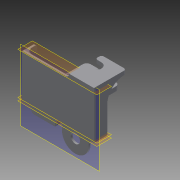
# Autodesk Inventor part: servo-holder
Saved by Autodesk Inventor 2014 (Build 180170000, 170)
## iProperties
Created: 2015-03-09
Part Number: servo-holder
Material: 一般
Document SubType Name: Modeling
Designer: Hideyuki Takei
Density: 1 g/cm^3
Appearance: 既定
Author: Hideyuki Takei
Autodesk Inventor part; units mm, degrees
ref_plane "YZ Plane" through (0, 0, 0) normal (1, 0, 0) x (0, 1, 0)
sketch "スケッチ2" plane through (0, 0, 0) normal (0, 1, 0) x (-1, 0, 0)
  line L0 (-8.8, 25.8) -> (27, 25.8)
  line L1 (27, 25.8) -> (27, 3.8)
  line L2 (27, 3.8) -> (-8.8, 3.8)
  line L3 (-8.8, 3.8) -> (-8.8, 25.8)
  line L4 (-8.8, 25.8) -> (-9.8, 25.8)
  line L5 (-9.8, 25.8) -> (-9.8, 3.8)
  line L6 (-9.8, 3.8) -> (-8.8, 3.8)
  line L7 (-8.8, 3.8) -> (-8.8, 25.8)
  line L8 (27, 25.8) -> (28, 25.8)
  line L9 (28, 25.8) -> (28, 3.8)
  line L10 (28, 3.8) -> (27, 3.8)
  line L11 (27, 3.8) -> (27, 25.8)
  point P0 (0, 0)
  dimension "d3" = 3.8
  dimension "d4" = 8.8
  dimension "d5" = 35.8
  dimension "d6" = 22
  dimension "d7" = 1
  dimension "d8" = 1
  dimension "d9" = 22
  dimension "d10" = 22
  constraints: 24 end point, 6 parallel, 3 horizontal, 3 perpendicular
  measures "d3" distance from line of point (0, 0) L2
  measures "d4" distance from line of point (0, 0) L3
  measures "d5" distance of L0.start L0.end
  measures "d6" distance of L2.end L0.start
  measures "d7" distance of L0.start L4.end
  measures "d8" distance of L0.end L8.end
  measures "d9" distance of L8.end L9.end
  measures "d10" distance of L4.end L5.end
extrude "押し出し2" add sketch "スケッチ2" along normal blind 7
ref_plane "作業平面4" through (0, 1, 0) normal (0, 1, 0) x (-1, 0, 0)
sketch "スケッチ3" plane through (0, 1, 0) normal (0, 1, 0) x (-1, 0, 0)
  line L0 (-8.8, 3.8) -> (27, 3.8)
  line L1 (27, 3.8) -> (27, 25.8)
  line L2 (27, 25.8) -> (-8.8, 25.8)
  line L3 (-8.8, 25.8) -> (-8.8, 3.8)
  point P0 (0, 0)
  dimension "d15" = 22
  dimension "d16" = 35.8
  dimension "d17" = 8.8
  dimension "d18" = 3.8
  constraints: 8 end point, 2 parallel, 1 horizontal, 1 perpendicular
  measures "d15" distance of L2.end L0.start
  measures "d16" distance of L1.end L2.end
  measures "d17" distance from line of point (0, 0) L3
  measures "d18" distance from line of point (0, 0) L0
extrude "押し出し3" cut sketch "スケッチ3" along normal up to next
fillet "フィレット3" radius 5 1 edges at (8.8, 1, 14.8)
sketch "スケッチ1" plane through (0, 0, 0) normal (0, 1, 0) x (-1, 0, 0)
  circle A0 centre (0, 0) radius 7
  dimension "d0" = 14
  constraints: 1 centre point, 1 coincident
  measures "d0" diameter of A0
extrude "押し出し1" add sketch "スケッチ1" along normal blind 1
fillet "フィレット4" radius 3 1 edges at (-27, 1, 14.8)
ref_plane "作業平面5" through (0, 0, 3.8) normal (0, 0, 1) x (1, 0, 0)
sketch "スケッチ4" plane through (0, 0, 3.8) normal (0, 0, 1) x (1, 0, 0)
  circle A0 centre (6.2, 3.6) radius 0.9
  line L0 (-7, 0) -> (7, 0) projected
  circle A1 centre (-24.9, 3.6) radius 0.9
  line L1 (9.8, 7) -> (4.3, 7)
  line L2 (4.3, 7) -> (4.3, 0)
  line L3 (4.3, 0) -> (9.8, 0)
  line L4 (9.8, 0) -> (9.8, 7)
  line L5 (9.8, 0) -> (9.8, 7) projected
  line L6 (-28, 7) -> (-22.7, 7)
  line L7 (-22.7, 7) -> (-22.7, 0)
  line L8 (-22.7, 0) -> (-28, 0)
  line L9 (-28, 0) -> (-28, 7)
  line L10 (-28, 0) -> (-28, 7) projected
  line L11 (-5.8788, 0) -> (-28, 0) projected
  point P0 (0, 0)
  point P1 (5.8788, 0)
  dimension "d27" = 3.6
  dimension "d28" = 6.2
  dimension "d29" = 1.8
  dimension "d30" = 1.8
  dimension "d31" = 3.6
  dimension "d32" = 24.9
  dimension "d33" = 5.5
  dimension "d34" = 7
  dimension "d35" = 0
  dimension "d36" = 0
  dimension "d37" = 5.3
  dimension "d38" = 0
  dimension "d39" = 0
  dimension "d40" = 7
  constraints: 16 end point, 4 parallel, 2 centre point, 2 horizontal, 2 perpendicular
  measures "d27" distance from line of L0 A0.centre
  measures "d28" horizontal distance of point (0, 0) A0.centre
  measures "d29" diameter of A0
  measures "d30" diameter of A1
  measures "d31" vertical distance of point (0, 0) A1.centre
  measures "d32" horizontal distance of A1.centre point (0, 0)
  measures "d33" distance of L1.start L1.end
  measures "d34" distance of L1.end L2.end
  measures "d35" distance between parallel lines of L0 L3
  measures "d36" distance between parallel lines of L5 L4
  measures "d37" distance of L6.start L6.end
  measures "d38" distance between parallel lines of L10 L9
  measures "d39" distance between parallel lines of L11 L8
  measures "d40" distance of L6.end L7.end
extrude "押し出し4" add sketch "スケッチ4" against normal blind 1
ref_plane "作業平面7" through (0, 0, 25.8) normal (0, 0, 1) x (1, 0, 0)
sketch "スケッチ6" plane through (0, 0, 25.8) normal (0, 0, 1) x (1, 0, 0)
  line L0 (9.8, 0) -> (-3.2, 0)
  line L1 (-3.2, 0) -> (-3.2, 17)
  line L2 (-3.2, 17) -> (9.8, 17)
  line L3 (9.8, 17) -> (9.8, 0)
  line L4 (9.8, 0) -> (9.8, 7) projected
  line L5 (-28, 0) -> (9.8, 0) projected
  circle A0 centre (0, 10.8) radius 2.9
  line L6 (0, 13.7) -> (-5.7401, 13.7)
  line L7 (-5.7401, 13.7) -> (-5.7401, 7.9)
  line L8 (-5.7401, 7.9) -> (0, 7.9)
  line L9 (0, 7.9) -> (0, 13.7)
  point P0 (0, 0)
  dimension "d58" = 5.8
  dimension "d54" = 0
  dimension "d55" = 0
  dimension "d56" = 13
  dimension "d57" = 17
  dimension "d59" = 9.8
  dimension "d60" = 10.8
  dimension "d61" = 5.8
  dimension "d62" = 2.9
  dimension "d63" = 5.7401
  constraints: 16 end point, 4 parallel, 2 horizontal, 2 perpendicular, 1 vertical alignment, 2 other
  measures "d54" distance between parallel lines of L4 L3
  measures "d55" distance between parallel lines of L5 L0
  measures "d56" distance of L1.end L2.end
  measures "d57" distance of L2.end L0.start
  measures "d59" distance from line of L3 point (0, 10.8)
  measures "d60" distance from line of L0 point (0, 10.8)
  measures "d61" distance of L6.end L7.end
  measures "d62" distance from line of L8 point (0, 10.8)
  measures "d63" distance of L6.start L6.end
extrude "押し出し5" add sketch "スケッチ6" along normal blind 2 contours L0 L1 L8 A0 L6 L2 L3 | L1 L6 A0 L8
sketch "スケッチ7" plane through (0, 0, 25.8) normal (0, 0, 1) x (1, 0, 0)
  line L0 (0, 13.7) -> (-9.1376, 13.7)
  line L1 (-9.1376, 13.7) -> (-9.1376, 7.9)
  line L2 (-9.1376, 7.9) -> (0, 7.9)
  line L3 (0, 7.9) -> (0, 13.7)
  line L4 (-3.2, 0) -> (9.8, 0) projected
  point P0 (0, 0)
  dimension "d66" = 5.8
  dimension "d67" = 7.9
  dimension "d68" = 0
  dimension "d69" = 9.1376
  constraints: 8 end point, 2 parallel, 1 horizontal, 1 perpendicular
  measures "d66" distance of L0.end L1.end
  measures "d67" distance between parallel lines of L4 L2
  measures "d68" distance from line of point (0, 0) L3
  measures "d69" distance of L0.start L0.end
extrude "押し出し6" cut sketch "スケッチ7" along normal blind 2
fillet "フィレット5" radius 3 1 edges at (4.3, 7, 3.3)
fillet "フィレット6" radius 1.2 5 edges at (-3.2, 17, 26.8) (-3.2, 13.7, 26.8) (9.8, 17, 26.8) (-3.2, 7.9, 26.8) (-27.5, 7, 25.8)
fillet "フィレット7" radius 2 1 edges at (-3.2, 0.5, 25.8)
fillet "フィレット8" radius 2 3 edges at (4.3, 1, 3.3) (-5.8788, 0.5, 3.8) (6.4156, 0.5, 2.8)
sketch "スケッチ8" plane through (0, 1, 0) normal (0, 1, 0) x (-1, 0, 0)
  circle A0 centre (0, 0) radius 2.5
  dimension "d76" = 5
  constraints: 1 centre point, 1 coincident
  measures "d76" diameter of A0
extrude "押し出し7" cut sketch "スケッチ8" against normal up to next
ref_plane "作業平面8" through (0, 0, 2.3) normal (0, 0, 1) x (1, 0, 0)
sketch "スケッチ9" plane through (0, 0, 2.3) normal (0, 0, 1) x (1, 0, 0)
  line L0 (-10.7, 34) -> (-22.7, 34)
  line L1 (-22.7, 34) -> (-22.7, 0)
  line L2 (-22.7, 0) -> (-10.7, 0)
  line L3 (-10.7, 0) -> (-10.7, 34)
  line L4 (-8.8182, 0) -> (-22.7, 0) projected
  line L5 (-22.7, 7) -> (-22.7, 0) projected
  point P0 (0, 0)
  dimension "d80" = 0
  dimension "d81" = 0
  dimension "d82" = 34
  dimension "d83" = 12
  constraints: 8 end point, 2 parallel, 1 horizontal, 1 perpendicular
  measures "d80" distance between parallel lines of L4 L2
  measures "d81" distance between parallel lines of L5 L1
  measures "d82" distance of L2.end L0.start
  measures "d83" distance of L0.start L0.end
extrude "押し出し8" add sketch "スケッチ9" against normal blind 2.3
sketch "スケッチ10" plane through (0, 0, 2.3) normal (0, 0, 1) x (1, 0, 0)
  line L0 (-10.7, 1) -> (-22.7, 1)
  line L1 (-22.7, 1) -> (-22.7, 0)
  line L2 (-22.7, 0) -> (-10.7, 0)
  line L3 (-10.7, 0) -> (-10.7, 1)
  line L4 (-10.7, 34) -> (-10.7, 0) projected
  line L5 (-10.7, 0) -> (-22.7, 0) projected
  point P0 (0, 0)
  dimension "d86" = 1
  dimension "d87" = 12
  dimension "d88" = 0
  dimension "d89" = 0
  constraints: 8 end point, 2 parallel, 1 horizontal, 1 perpendicular
  measures "d86" distance of L2.end L0.start
  measures "d87" distance of L1.end L2.end
  measures "d88" distance between parallel lines of L4 L3
  measures "d89" distance between parallel lines of L5 L2
extrude "押し出し9" add sketch "スケッチ10" along normal up to next
sketch "スケッチ11" plane through (0, 0, 3.8) normal (0, 0, 1) x (1, 0, 0)
  line L0 (-22.7, 34) -> (-28, 34)
  line L1 (-28, 34) -> (-28, 7)
  line L2 (-28, 7) -> (-22.7, 7)
  line L3 (-22.7, 7) -> (-22.7, 34)
  line L4 (-22.7, 1) -> (-22.7, 0) projected
  line L5 (-28, 0) -> (-28, 7) projected
  line L6 (-28, 7) -> (-22.7, 7) projected
  line L7 (-22.7, 34) -> (-10.7, 34) projected
  point P0 (0, 0)
  dimension "d93" = 0
  dimension "d94" = 0
  dimension "d95" = 0
  dimension "d108" = 5.3
  constraints: 8 end point, 2 parallel, 1 horizontal, 1 perpendicular
  measures "d93" distance between parallel lines of L5 L1
  measures "d94" distance between parallel lines of L6 L2
  measures "d95" distance between parallel lines of L7 L0
  measures "d108" distance between parallel lines of L1 L3
extrude "押し出し10" add sketch "スケッチ11" against normal blind 1
sketch "スケッチ12" plane through (0, 0, 2.8) normal (0, 0, -1) x (-1, 0, 0)
  line L0 (22.7, 34) -> (22.7, 0) projected
  line L1 (22.7, 1) -> (22.7, 0) projected
  line L2 (22.7, 0) -> (28, 0) projected
  line L3 (22.7, 34) -> (23.2, 34)
  line L4 (23.2, 34) -> (23.2, 0)
  line L5 (23.2, 0) -> (22.7, 0)
  line L6 (22.7, 0) -> (22.7, 34)
  point P0 (0, 0)
  dimension "d98" = 0.5
  constraints: 8 end point, 2 parallel, 1 horizontal, 1 perpendicular, 1 point on line
  measures "d98" distance of L0.start L3.end
extrude "押し出し11" add sketch "スケッチ12" along normal blind 2.8
fillet "フィレット13" radius 1.5 2 edges at (-23.2, 17, 0) (-23.2, 17, 2.8)
fillet "フィレット9" radius 19 1 edges at (-27.5, 7, 3.8)
sketch "スケッチ13" plane through (0, 0, 2.8) normal (0, 0, -1) x (-1, 0, 0)
  arc A0 (24, 3.6) -> (24, 3.6) centre (24.9, 3.6) ccw projected
  circle A1 centre (24.9, 3.6) radius 1.6
  point P0 (0, 0)
  dimension "d103" = 3.2
  constraints: 1 centre point, 1 coincident
  measures "d103" diameter of A1
extrude "押し出し12" cut sketch "スケッチ13" along normal blind 2.5 contours A0 | A1
fillet "フィレット11" radius 2 2 edges at (-28, 34, 3.3) (-10.7, 34, 1.15)
fillet "フィレット14" radius 9 1 edges at (9.3, 7, 25.8)
fillet "フィレット15" radius 1.5 1 edges at (-10.7, 0.5, 3.8)
sketch "スケッチ14" plane through (-22.7, 1, 2.3) normal (1, 0, 0) x (0, 0, -1)
  line L0 (0, 33) -> (0, 0) projected
  line L1 (-1.5, 33) -> (0, 33)
  line L2 (0, 33) -> (0, 28)
  line L3 (0, 28) -> (-1.5, 28)
  line L4 (-1.5, 28) -> (-1.5, 33)
  point P0 (2.3, -1)
  dimension "d112" = 5
  constraints: 8 end point, 2 parallel, 1 horizontal, 1 perpendicular, 1 point on line
  measures "d112" distance of L3.end L1.start
extrude "押し出し13" add sketch "スケッチ14" along normal blind 2
fillet "フィレット16" radius 1.5 1 edges at (-20.7, 31.5, 3.8)
sketch "スケッチ16" plane through (0, 0, 2.3) normal (0, 0, 1) x (1, 0, 0)
  circle A0 centre (-16, 27.8) radius 2
  line L0 (-3.2, 0) -> (9.8, 0) projected
  point P0 (0, 0)
  point P1 (0, 10.8)
  dimension "d116" = 4
  dimension "d117" = 10.8
  dimension "d118" = 16
  dimension "d119" = 17
  constraints: 1 centre point
  measures "d116" diameter of A0
  measures "d117" distance from line of L0 point (0, 10.8)
  measures "d118" horizontal distance of point (0, 10.8) A0.centre
  measures "d119" vertical distance of A0.centre point (0, 10.8)
extrude "押し出し14" cut sketch "スケッチ16" against normal up to next
equation "\"d62\" = 0.5 * d61"
